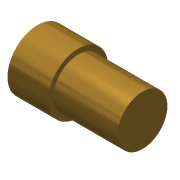
# Autodesk Inventor part: Motor
Saved by Autodesk Inventor 2016 (Build 200138000, 138)
## iProperties
Created: 2015-05-19
Part Number: Motor
Material: Generic
Document SubType Name: Modeling
Designer: CHUNGBK
Density: 3.43259 g/cm^3
Appearance: Brass - Satin
Mass: 500 g
Surface Area: 171.804 cm^2
Volume: 145.663 cm^3
Author: CHUNGBK
Autodesk Inventor part; units mm, degrees
ref_plane "YZ Plane" through (0, 0, 0) normal (1, 0, 0) x (0, 1, 0)
ref_plane "XZ Plane" through (0, 0, 0) normal (0, 1, 0) x (-1, 0, 0)
ref_plane "XY Plane" through (0, 0, 0) normal (0, 0, 1) x (1, 0, 0)
sketch "Sketch1" plane through (0, 0, 0) normal (1, 0, 0) x (0, 1, 0)
  circle A0 centre (0, 0) radius 25.4
  dimension "d0" = 50.8
  constraints: 1 centre point, 1 coincident
  measures "d0" diameter of A0
extrude "Extrusion1" add sketch "Sketch1" along normal blind 34.544
sketch "Sketch2" plane through (34.544, 0, 0) normal (1, 0, 0) x (0, 0, -1)
  circle A0 centre (0, 0) radius 21.082
  dimension "d3" = 42.164
  constraints: 1 centre point, 1 coincident
  measures "d3" diameter of A0
extrude "Extrusion2" add sketch "Sketch2" along normal blind 54.61
sketch "Sketch3" plane through (0, 0, 0) normal (-1, 0, 0) x (0, 0, 1)
  circle A0 centre (0, 8.3566) radius 3.175
  line L0 (0, 0) -> (0, 8.3566) construction
  circle A1 centre (0, 0) radius 25.4 projected
  dimension "d9" = 6.35
  dimension "d10" = 8.3566
  constraints: 2 end point, 1 centre point, 1 coincident, 1 vertical
  measures "d9" diameter of A0
  measures "d10" distance of L0.start L0.end
extrude "Extrusion3" cut sketch "Sketch3" against normal blind 19.05 contours A0
body "Solid1"
